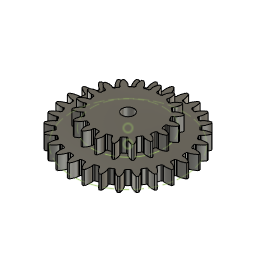
front axle gear v4 (Autodesk Fusion 360 design; units mm, degrees)
description: Spur Gear; Module: 2.0; Num Teeth: 28; Pressure Angle: 20.0; Backlash: 1.00 mm
description: Spur Gear; Module: 2.0; Num Teeth: 18; Pressure Angle: 20.0; Backlash: 1.00 mm
Autodesk Fusion 360 part; units mm, degrees
sketch "Sketch1" plane through (0, 0, 0) normal (0, 0, 1) x (1, 0, 0) in component "Spur Gear (28 teeth)"
  circle A0 centre (0, 0) radius 25.5492
  circle A1 centre (0, 0) radius 3
extrude "Extrude1" add sketch "Sketch1" along normal blind 7 makes body 1 in component "Spur Gear (28 teeth)"
sketch "Sketch2" plane through (0, 0, 0) normal (0, 0, 1) x (1, 0, 0) in component "Spur Gear (28 teeth)"
  spline S0 degree 5 poles (26.2607, -1.6322) (26.2715, -1.6329) (26.2931, -1.634) (26.3254, -1.6348) (26.3686, -1.6345) (26.4225, -1.632) (26.4765, -1.6281) (26.5306, -1.6233) (26.5846, -1.618) (26.6386, -1.6123) (26.6927, -1.6063) (26.7467, -1.5999) (26.8008, -1.5928) (26.8548, -1.5851) (26.9089, -1.5767) (26.9629, -1.5676) (27.0169, -1.5579) (27.0709, -1.5478) (27.1249, -1.5372) (27.1789, -1.5263) (27.2329, -1.515) (27.2868, -1.5033) (27.3407, -1.4912) (27.3946, -1.4786) (27.4485, -1.4656) (27.5024, -1.4522) (27.5562, -1.4384) (27.61, -1.4242) (27.6638, -1.4097) (27.7176, -1.3948) (27.7714, -1.3795) (27.8251, -1.3639) (27.8788, -1.348) (27.9324, -1.3317) (27.9861, -1.315) (28.0397, -1.298) (28.0933, -1.2807) (28.1468, -1.2631) (28.2003, -1.2451) (28.2538, -1.2269) (28.3073, -1.2083) (28.3607, -1.1894) (28.414, -1.1702) (28.4674, -1.1507) (28.5207, -1.1308) (28.574, -1.1107) (28.6272, -1.0903) (28.6804, -1.0696) (28.7336, -1.0486) (28.7867, -1.0273) (28.8398, -1.0058) (28.8928, -0.9839) (28.9458, -0.9618) (28.9988, -0.9394) (29.0517, -0.9167) (29.1046, -0.8937) (29.1574, -0.8705) (29.2102, -0.847) (29.2629, -0.8232) (29.3156, -0.7992) (29.3683, -0.7749) (29.4209, -0.7503) (29.4735, -0.7255) (29.526, -0.7004) (29.5785, -0.6751) (29.6309, -0.6495) (29.6832, -0.6236) (29.7356, -0.5975) (29.7878, -0.5711) (29.8401, -0.5445) (29.8922, -0.5177) (29.9339, -0.496) (29.9652, -0.4796) (29.986, -0.4686) (29.9964, -0.4631) knots 0 0 0 0 0 0 0.01428571 0.02857143 0.04285714 0.05714286 0.07142857 0.08571429 0.1 0.11428571 0.12857143 0.14285714 0.15714286 0.17142857 0.18571429 0.2 0.21428571 0.22857143 0.24285714 0.25714286 0.27142857 0.28571429 0.3 0.31428571 0.32857143 0.34285714 0.35714286 0.37142857 0.38571429 0.4 0.41428571 0.42857143 0.44285714 0.45714286 0.47142857 0.48571429 0.5 0.51428571 0.52857143 0.54285714 0.55714286 0.57142857 0.58571429 0.6 0.61428571 0.62857143 0.64285714 0.65714286 0.67142857 0.68571429 0.7 0.71428571 0.72857143 0.74285714 0.75714286 0.77142857 0.78571429 0.8 0.81428571 0.82857143 0.84285714 0.85714286 0.87142857 0.88571429 0.9 0.91428571 0.92857143 0.94285714 0.95714286 0.97142857 0.98571429 1 1 1 1 1 1
  spline S1 degree 5 poles (26.2607, 1.6322) (26.2715, 1.6329) (26.2931, 1.634) (26.3254, 1.6348) (26.3686, 1.6345) (26.4225, 1.632) (26.4765, 1.6281) (26.5306, 1.6233) (26.5846, 1.618) (26.6386, 1.6123) (26.6927, 1.6063) (26.7467, 1.5999) (26.8008, 1.5928) (26.8548, 1.5851) (26.9089, 1.5767) (26.9629, 1.5676) (27.0169, 1.5579) (27.0709, 1.5478) (27.1249, 1.5372) (27.1789, 1.5263) (27.2329, 1.515) (27.2868, 1.5033) (27.3407, 1.4912) (27.3946, 1.4786) (27.4485, 1.4656) (27.5024, 1.4522) (27.5562, 1.4384) (27.61, 1.4242) (27.6638, 1.4097) (27.7176, 1.3948) (27.7714, 1.3795) (27.8251, 1.3639) (27.8788, 1.348) (27.9324, 1.3317) (27.9861, 1.315) (28.0397, 1.298) (28.0933, 1.2807) (28.1468, 1.2631) (28.2003, 1.2451) (28.2538, 1.2269) (28.3073, 1.2083) (28.3607, 1.1894) (28.414, 1.1702) (28.4674, 1.1507) (28.5207, 1.1308) (28.574, 1.1107) (28.6272, 1.0903) (28.6804, 1.0696) (28.7336, 1.0486) (28.7867, 1.0273) (28.8398, 1.0058) (28.8928, 0.9839) (28.9458, 0.9618) (28.9988, 0.9394) (29.0517, 0.9167) (29.1046, 0.8937) (29.1574, 0.8705) (29.2102, 0.847) (29.2629, 0.8232) (29.3156, 0.7992) (29.3683, 0.7749) (29.4209, 0.7503) (29.4735, 0.7255) (29.526, 0.7004) (29.5785, 0.6751) (29.6309, 0.6495) (29.6832, 0.6236) (29.7356, 0.5975) (29.7878, 0.5711) (29.8401, 0.5445) (29.8922, 0.5177) (29.9339, 0.496) (29.9652, 0.4796) (29.986, 0.4686) (29.9964, 0.4631) knots 0 0 0 0 0 0 0.01428571 0.02857143 0.04285714 0.05714286 0.07142857 0.08571429 0.1 0.11428571 0.12857143 0.14285714 0.15714286 0.17142857 0.18571429 0.2 0.21428571 0.22857143 0.24285714 0.25714286 0.27142857 0.28571429 0.3 0.31428571 0.32857143 0.34285714 0.35714286 0.37142857 0.38571429 0.4 0.41428571 0.42857143 0.44285714 0.45714286 0.47142857 0.48571429 0.5 0.51428571 0.52857143 0.54285714 0.55714286 0.57142857 0.58571429 0.6 0.61428571 0.62857143 0.64285714 0.65714286 0.67142857 0.68571429 0.7 0.71428571 0.72857143 0.74285714 0.75714286 0.77142857 0.78571429 0.8 0.81428571 0.82857143 0.84285714 0.85714286 0.87142857 0.88571429 0.9 0.91428571 0.92857143 0.94285714 0.95714286 0.97142857 0.98571429 1 1 1 1 1 1
  arc A0 (29.9964, -0.4631) -> (29.9964, 0.4631) centre (0, 0) ccw
  line L0 (25.49, -1.585) -> (26.2607, -1.6322)
  line L1 (25.49, 1.585) -> (26.2607, 1.6322)
  line L2 (25.49, -1.585) -> (25.49, 1.585)
  point P0 (26.5252, -1.6236)
  point P1 (26.791, -1.594)
  point P2 (27.0574, -1.5502)
  point P3 (27.3244, -1.4948)
  point P4 (27.5918, -1.429)
  point P5 (27.8594, -1.3537)
  point P6 (28.1271, -1.2696)
  point P7 (28.3948, -1.1771)
  point P8 (28.6624, -1.0766)
  point P9 (28.9299, -0.9684)
  point P10 (29.1971, -0.8528)
  point P11 (29.464, -0.7299)
  point P12 (29.7305, -0.6)
  point P13 (26.5252, 1.6236)
  point P14 (26.791, 1.594)
  point P15 (27.0574, 1.5502)
  point P16 (27.3244, 1.4948)
  point P17 (27.5918, 1.429)
  point P18 (27.8594, 1.3537)
  point P19 (28.1271, 1.2696)
  point P20 (28.3948, 1.1771)
  point P21 (28.6624, 1.0766)
  point P22 (28.9299, 0.9684)
  point P23 (29.1971, 0.8528)
  point P24 (29.464, 0.7299)
  point P25 (29.7305, 0.6)
extrude "Extrude2" add sketch "Sketch2" along normal blind 7 bodies 1 in component "Spur Gear (28 teeth)"
fillet "Fillet1" radius 0.5 2 edges at (25.5, -1.5856, 3.5) (25.5, 1.5856, 3.5) on bodies 1 in component "Spur Gear (28 teeth)"
pattern_circular "C-Pattern1" count 28 over 360 about axis through (0, 0, 0) along (0, 0, 1) of "Extrude2", "Fillet1" in component "Spur Gear (28 teeth)"
sketch "Sketch3" plane through (0, 0, 0) normal (0, 0, 1) x (1, 0, 0) in component "Spur Gear (28 teeth)"
  circle A0 centre (0, 0) radius 28 construction
sketch "Sketch1 (2)" plane through (0, 0, 0) normal (0, 0, 1) x (1, 0, 0) in component "Spur Gear (18 teeth)"
  circle A0 centre (0, 0) radius 15.5492
  circle A1 centre (0, 0) radius 3
extrude "Extrude1'" add sketch "Sketch1 (2)" along normal blind 7 separate body makes body 2 in component "Spur Gear (18 teeth)"
sketch "Sketch2 (2)" plane through (0, 0, 0) normal (0, 0, 1) x (1, 0, 0) in component "Spur Gear (18 teeth)"
  spline S0 degree 5 poles (16.8486, -1.4913) (16.8576, -1.4921) (16.8758, -1.4934) (16.9029, -1.4947) (16.9392, -1.495) (16.9846, -1.4934) (17.0301, -1.4904) (17.0756, -1.4866) (17.1212, -1.4823) (17.1668, -1.4776) (17.2123, -1.4726) (17.2579, -1.4672) (17.3035, -1.4612) (17.3491, -1.4545) (17.3947, -1.4471) (17.4403, -1.4391) (17.486, -1.4305) (17.5316, -1.4215) (17.5772, -1.4121) (17.6227, -1.4023) (17.6683, -1.3922) (17.7139, -1.3816) (17.7594, -1.3706) (17.805, -1.3592) (17.8505, -1.3474) (17.896, -1.3352) (17.9415, -1.3226) (17.987, -1.3096) (18.0324, -1.2962) (18.0778, -1.2825) (18.1232, -1.2685) (18.1686, -1.2541) (18.214, -1.2394) (18.2593, -1.2243) (18.3046, -1.2089) (18.3498, -1.1931) (18.3951, -1.177) (18.4403, -1.1606) (18.4855, -1.1439) (18.5306, -1.1268) (18.5757, -1.1095) (18.6208, -1.0918) (18.6658, -1.0739) (18.7108, -1.0556) (18.7558, -1.037) (18.8007, -1.0181) (18.8456, -0.999) (18.8904, -0.9795) (18.9352, -0.9598) (18.98, -0.9397) (19.0247, -0.9194) (19.0694, -0.8988) (19.114, -0.8779) (19.1586, -0.8567) (19.2031, -0.8353) (19.2476, -0.8135) (19.292, -0.7916) (19.3364, -0.7693) (19.3808, -0.7468) (19.4251, -0.724) (19.4693, -0.7009) (19.5135, -0.6776) (19.5576, -0.654) (19.6017, -0.6301) (19.6457, -0.606) (19.6897, -0.5816) (19.7336, -0.557) (19.7775, -0.5321) (19.8213, -0.507) (19.865, -0.4816) (19.9087, -0.4559) (19.9436, -0.4352) (19.9698, -0.4196) (19.9872, -0.4091) (19.9959, -0.4039) knots 0 0 0 0 0 0 0.01428571 0.02857143 0.04285714 0.05714286 0.07142857 0.08571429 0.1 0.11428571 0.12857143 0.14285714 0.15714286 0.17142857 0.18571429 0.2 0.21428571 0.22857143 0.24285714 0.25714286 0.27142857 0.28571429 0.3 0.31428571 0.32857143 0.34285714 0.35714286 0.37142857 0.38571429 0.4 0.41428571 0.42857143 0.44285714 0.45714286 0.47142857 0.48571429 0.5 0.51428571 0.52857143 0.54285714 0.55714286 0.57142857 0.58571429 0.6 0.61428571 0.62857143 0.64285714 0.65714286 0.67142857 0.68571429 0.7 0.71428571 0.72857143 0.74285714 0.75714286 0.77142857 0.78571429 0.8 0.81428571 0.82857143 0.84285714 0.85714286 0.87142857 0.88571429 0.9 0.91428571 0.92857143 0.94285714 0.95714286 0.97142857 0.98571429 1 1 1 1 1 1
  spline S1 degree 5 poles (16.8486, 1.4913) (16.8576, 1.4921) (16.8758, 1.4934) (16.9029, 1.4947) (16.9392, 1.495) (16.9846, 1.4934) (17.0301, 1.4904) (17.0756, 1.4866) (17.1212, 1.4823) (17.1668, 1.4776) (17.2123, 1.4726) (17.2579, 1.4672) (17.3035, 1.4612) (17.3491, 1.4545) (17.3947, 1.4471) (17.4403, 1.4391) (17.486, 1.4305) (17.5316, 1.4215) (17.5772, 1.4121) (17.6227, 1.4023) (17.6683, 1.3922) (17.7139, 1.3816) (17.7594, 1.3706) (17.805, 1.3592) (17.8505, 1.3474) (17.896, 1.3352) (17.9415, 1.3226) (17.987, 1.3096) (18.0324, 1.2962) (18.0778, 1.2825) (18.1232, 1.2685) (18.1686, 1.2541) (18.214, 1.2394) (18.2593, 1.2243) (18.3046, 1.2089) (18.3498, 1.1931) (18.3951, 1.177) (18.4403, 1.1606) (18.4855, 1.1439) (18.5306, 1.1268) (18.5757, 1.1095) (18.6208, 1.0918) (18.6658, 1.0739) (18.7108, 1.0556) (18.7558, 1.037) (18.8007, 1.0181) (18.8456, 0.999) (18.8904, 0.9795) (18.9352, 0.9598) (18.98, 0.9397) (19.0247, 0.9194) (19.0694, 0.8988) (19.114, 0.8779) (19.1586, 0.8567) (19.2031, 0.8353) (19.2476, 0.8135) (19.292, 0.7916) (19.3364, 0.7693) (19.3808, 0.7468) (19.4251, 0.724) (19.4693, 0.7009) (19.5135, 0.6776) (19.5576, 0.654) (19.6017, 0.6301) (19.6457, 0.606) (19.6897, 0.5816) (19.7336, 0.557) (19.7775, 0.5321) (19.8213, 0.507) (19.865, 0.4816) (19.9087, 0.4559) (19.9436, 0.4352) (19.9698, 0.4196) (19.9872, 0.4091) (19.9959, 0.4039) knots 0 0 0 0 0 0 0.01428571 0.02857143 0.04285714 0.05714286 0.07142857 0.08571429 0.1 0.11428571 0.12857143 0.14285714 0.15714286 0.17142857 0.18571429 0.2 0.21428571 0.22857143 0.24285714 0.25714286 0.27142857 0.28571429 0.3 0.31428571 0.32857143 0.34285714 0.35714286 0.37142857 0.38571429 0.4 0.41428571 0.42857143 0.44285714 0.45714286 0.47142857 0.48571429 0.5 0.51428571 0.52857143 0.54285714 0.55714286 0.57142857 0.58571429 0.6 0.61428571 0.62857143 0.64285714 0.65714286 0.67142857 0.68571429 0.7 0.71428571 0.72857143 0.74285714 0.75714286 0.77142857 0.78571429 0.8 0.81428571 0.82857143 0.84285714 0.85714286 0.87142857 0.88571429 0.9 0.91428571 0.92857143 0.94285714 0.95714286 0.97142857 0.98571429 1 1 1 1 1 1
  arc A0 (19.9959, -0.4039) -> (19.9959, 0.4039) centre (0, 0) ccw
  line L0 (15.4787, -1.3709) -> (16.8486, -1.4913)
  line L1 (15.4787, 1.3709) -> (16.8486, 1.4913)
  line L2 (15.4787, -1.3709) -> (15.4787, 1.3709)
  point P0 (17.0702, -1.4869)
  point P1 (17.2935, -1.4624)
  point P2 (17.5179, -1.4242)
  point P3 (17.7429, -1.3746)
  point P4 (17.9684, -1.3148)
  point P5 (18.1942, -1.2457)
  point P6 (18.4203, -1.1678)
  point P7 (18.6463, -1.0816)
  point P8 (18.8722, -0.9874)
  point P9 (19.0979, -0.8854)
  point P10 (19.3232, -0.7759)
  point P11 (19.5481, -0.659)
  point P12 (19.7724, -0.535)
  point P13 (17.0702, 1.4869)
  point P14 (17.2935, 1.4624)
  point P15 (17.5179, 1.4242)
  point P16 (17.7429, 1.3746)
  point P17 (17.9684, 1.3148)
  point P18 (18.1942, 1.2457)
  point P19 (18.4203, 1.1678)
  point P20 (18.6463, 1.0816)
  point P21 (18.8722, 0.9874)
  point P22 (19.0979, 0.8854)
  point P23 (19.3232, 0.7759)
  point P24 (19.5481, 0.659)
  point P25 (19.7724, 0.535)
extrude "Extrude2'" add sketch "Sketch2 (2)" along normal blind 7 bodies 2 in component "Spur Gear (18 teeth)"
fillet "Fillet1'" radius 0.5 2 edges at (15.4886, -1.3718, 3.5) (15.4886, 1.3718, 3.5) on bodies 2 in component "Spur Gear (18 teeth)"
pattern_circular "C-Pattern1'" count 18 over 360 about axis through (0, 0, 0) along (0, 0, 1) of "Extrude2'", "Fillet1'" in component "Spur Gear (18 teeth)"
sketch "Sketch3 (2)" plane through (0, 0, 0) normal (0, 0, 1) x (1, 0, 0) in component "Spur Gear (18 teeth)"
  circle A0 centre (0, 0) radius 18 construction
combine "Combine1" operation add target body 2 tool bodies 1 body 1 seen with x (1, 0, 0) y (0, 1, 0) z (0, 0, 1) at (0, 0, -7) in component "Spur Gear (18 teeth)"
component "Spur Gear (28 teeth)" placed x (1, 0, 0) y (0, 1, 0) z (0, 0, 1) at (0, 0, 0)
component "Spur Gear (18 teeth)" placed x (1, 0, 0) y (0, 1, 0) z (0, 0, 1) at (0, 0, 7)
